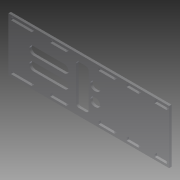
# Autodesk Inventor part: Top_plate2
Saved by Autodesk Inventor 2015 (Build 190159000, 159)
## iProperties
Created: 2015-06-18
Part Number: Top_plate2
Material: Generic
Document SubType Name: Modeling
Designer: Openlab
Density: 1 g/cm^3
Appearance: Polycarbonate - Clear
Author: Openlab
Autodesk Inventor part; units mm, degrees
ref_plane "YZ Plane" through (0, 0, 0) normal (1, 0, 0) x (0, 1, 0)
ref_plane "XZ Plane" through (0, 0, 0) normal (0, 1, 0) x (-1, 0, 0)
ref_plane "XY Plane" through (0, 0, 0) normal (0, 0, 1) x (1, 0, 0)
sketch "Sketch1" plane through (0, 0, 0) normal (0, 1, 0) x (-1, 0, 0)
  line L0 (37.25, -2.25) -> (24.75, -2.25) construction
  line L1 (24.75, -2.25) -> (24.75, -14.75) construction
  line L2 (24.75, -14.75) -> (37.25, -14.75) construction
  line L3 (37.25, -14.75) -> (37.25, -2.25) construction
  line L4 (56.9183, -8.5) -> (8.3915, -8.5) construction
  line L5 (0, -17) -> (105, -17) construction
  line L6 (0, 0) -> (0, -51) construction
  line L7 (0, -34) -> (105, -34) construction
  line L8 (105, -51) -> (105, 0) construction
  line L9 (31, 19) -> (31, -51) construction
  line L10 (56.8064, -25.5) -> (17, -25.5) construction
  line L11 (24.75, -19.25) -> (24.75, -31.75) construction
  line L12 (37.25, -19.25) -> (24.75, -19.25) construction
  line L13 (37.25, -31.75) -> (37.25, -19.25) construction
  line L14 (24.75, -31.75) -> (37.25, -31.75) construction
  line L15 (24.75, -36.25) -> (24.75, -48.75) construction
  line L16 (37.25, -36.25) -> (24.75, -36.25) construction
  line L17 (37.25, -48.75) -> (37.25, -36.25) construction
  line L18 (24.75, -48.75) -> (37.25, -48.75) construction
  line L19 (56.3008, -42.5) -> (16.5498, -42.5) construction
  arc A0 (53.45, -12) -> (53.45, -22) centre (53.45, -17) ccw
  arc A1 (92, -22) -> (92, -12) centre (92, -17) ccw
  arc A2 (53.45, -29) -> (53.45, -39) centre (53.45, -34) ccw
  arc A3 (92, -39) -> (92, -29) centre (92, -34) ccw
  line L20 (53.45, -12) -> (92, -12)
  line L21 (53.45, -22) -> (92, -22)
  line L22 (53.45, -29) -> (92, -29)
  line L23 (53.45, -39) -> (92, -39)
  arc A4 (16.15, -39) -> (16.15, -29) centre (16.15, -34) ccw
  line L24 (103.5, -49.5) -> (103.5, -1.5) construction
  line L25 (1.5, -1.5) -> (1.5, -49.5) construction
  arc A5 (14, -29) -> (14, -39) centre (14, -34) ccw
  arc A6 (14, -12) -> (14, -22) centre (14, -17) ccw
  line L26 (16.15, -39) -> (14, -39)
  line L27 (14, -29) -> (16.15, -29)
  line L28 (14, -22) -> (16.15, -22)
  line L29 (16.15, -12) -> (14, -12)
  arc A7 (16.15, -22) -> (16.15, -12) centre (16.15, -17) ccw
  arc A8 (96.5, -51) -> (93, -47.5) centre (93, -51) ccw construction
  arc A9 (53.45, -47.5) -> (49.95, -51) centre (53.45, -51) ccw construction
  arc A10 (97.7697, -49.5) -> (93, -46) centre (93, -51) ccw construction
  line L30 (93, -46) -> (53.45, -46) construction
  line L31 (96.5, -51) -> (105, -51) construction
  line L32 (93, -47.5) -> (53.45, -47.5) construction
  line L33 (105, -49.5) -> (97.7697, -49.5) construction
  arc A11 (53.45, -46) -> (48.6803, -49.5) centre (53.45, -51) ccw construction
  arc A12 (48.6803, -1.5) -> (53.45, -5) centre (53.45, 0) ccw construction
  arc A13 (49.95, 0) -> (53.45, -3.5) centre (53.45, 0) ccw construction
  line L34 (93, -3.5) -> (53.45, -3.5) construction
  line L35 (93, -5) -> (53.45, -5) construction
  line L36 (97.7697, -1.5) -> (105, -1.5) construction
  line L37 (105, 0) -> (96.5, 0) construction
  arc A14 (93, -3.5) -> (96.5, 0) centre (93, 0) ccw construction
  arc A15 (93, -5) -> (97.7697, -1.5) centre (93, 0) ccw construction
  arc A16 (16.65, -51) -> (13.15, -47.5) centre (13.15, -51) ccw construction
  arc A17 (12, -47.5) -> (8.5, -51) centre (12, -51) ccw construction
  line L38 (13.15, -46) -> (12, -46) construction
  line L39 (13.15, -47.5) -> (12, -47.5) construction
  arc A18 (12, -46) -> (7.2303, -49.5) centre (12, -51) ccw construction
  arc A19 (17.9197, -49.5) -> (13.15, -46) centre (13.15, -51) ccw construction
  line L40 (48.6803, -49.5) -> (17.9197, -49.5) construction
  line L41 (7.2303, -49.5) -> (0, -49.5) construction
  line L42 (0, -51) -> (8.5, -51) construction
  line L43 (16.65, -51) -> (49.95, -51) construction
  line L44 (13.15, -5) -> (12, -5) construction
  line L45 (13.15, -3.5) -> (12, -3.5) construction
  arc A20 (8.5, 0) -> (12, -3.5) centre (12, 0) ccw construction
  arc A21 (13.15, -3.5) -> (16.65, 0) centre (13.15, 0) ccw construction
  arc A22 (7.2303, -1.5) -> (12, -5) centre (12, 0) ccw construction
  arc A23 (13.15, -5) -> (17.9197, -1.5) centre (13.15, 0) ccw construction
  line L46 (49.95, 0) -> (16.65, 0) construction
  line L47 (8.5, 0) -> (0, 0) construction
  line L48 (0, -1.5) -> (7.2303, -1.5) construction
  line L49 (17.9197, -1.5) -> (48.6803, -1.5) construction
  line L50 (-74, 2) -> (-74, -53)
  line L51 (120, -53) -> (120, 2)
  arc A24 (38.75, -4.25) -> (35.25, -0.75) centre (35.25, -4.25) ccw
  arc A25 (26.75, -0.75) -> (23.25, -4.25) centre (26.75, -4.25) ccw
  arc A26 (35.25, -50.25) -> (38.75, -46.75) centre (35.25, -46.75) ccw
  arc A27 (23.25, -46.75) -> (26.75, -50.25) centre (26.75, -46.75) ccw
  line L52 (38.75, -4.25) -> (38.75, -46.75)
  line L53 (35.25, -0.75) -> (26.75, -0.75)
  line L54 (23.25, -4.25) -> (23.25, -46.75)
  line L55 (26.75, -50.25) -> (35.25, -50.25)
  line L56 (120, -53) -> (120, -56)
  line L57 (-74, -56) -> (-74, -53)
  line L58 (120, 2) -> (120, 5)
  line L59 (-74, 5) -> (-74, 2)
  line L60 (51, -56) -> (51, -53)
  line L61 (11, -56) -> (11, -53)
  line L62 (71, -56) -> (71, -53)
  line L63 (94, -53) -> (94, -56)
  line L64 (-9, -53) -> (-9, -56)
  line L65 (-59, -56) -> (-59, -53)
  line L66 (94, 2) -> (94, 5)
  line L67 (71, 2) -> (71, 5)
  line L68 (51, 2) -> (51, 5)
  line L69 (11, 2) -> (11, 5)
  line L70 (-9, 2) -> (-9, 5)
  line L71 (-59, 2) -> (-59, 5)
  line L72 (120, -56) -> (123, -56)
  line L73 (123, -56) -> (123, 5)
  line L74 (123, 5) -> (120, 5)
  line L75 (-74, 5) -> (-77, 5)
  line L76 (-77, 5) -> (-77, -56)
  line L77 (-77, -56) -> (-74, -56)
  line L78 (123, -56) -> (123, -59)
  line L79 (123, -59) -> (-77, -59)
  line L80 (-77, -59) -> (-77, -56)
  line L81 (123, 5) -> (123, 8)
  line L82 (123, 8) -> (-77, 8)
  line L83 (-77, 8) -> (-77, 5)
  line L84 (120, -56) -> (94, -56)
  line L85 (71, -56) -> (51, -56)
  line L86 (11, -56) -> (-9, -56)
  line L87 (-59, -56) -> (-74, -56)
  line L88 (-59, -53) -> (-74, -53)
  line L89 (-9, -53) -> (11, -53)
  line L90 (51, -53) -> (71, -53)
  line L91 (94, -53) -> (120, -53)
  line L92 (120, 5) -> (94, 5)
  line L93 (120, 2) -> (94, 2)
  line L94 (71, 2) -> (51, 2)
  line L95 (71, 5) -> (51, 5)
  line L96 (11, 2) -> (-9, 2)
  line L97 (11, 5) -> (-9, 5)
  line L98 (-59, 2) -> (-74, 2)
  line L99 (-59, 5) -> (-74, 5)
  line L100 (-24, -53) -> (-39, -53)
  line L101 (-39, -53) -> (-39, -56)
  line L102 (-39, -56) -> (-24, -56)
  line L103 (-24, -56) -> (-24, -53)
  line L104 (-24, 5) -> (-39, 5)
  line L105 (-39, 5) -> (-39, 2)
  line L106 (-39, 2) -> (-24, 2)
  line L107 (-24, 2) -> (-24, 5)
  point P0 (31, -8.5)
  point P1 (31, -42.5)
  point P2 (31, -25.5)
  dimension "d0" = 12.5
  dimension "d1" = 12.5
  dimension "d2" = 17
  dimension "d3" = 31
  dimension "d4" = 105
  dimension "d5" = 17
  dimension "d6" = 17
  dimension "d7" = 10
  dimension "d8" = 1.5
  dimension "d9" = 1.5
  dimension "d10" = 5
  dimension "d11" = 1.5
  dimension "d12" = 1.5
  dimension "d13" = 1.5
  dimension "d14" = 17
  dimension "d15" = 17
  dimension "d16" = 12
  dimension "d17" = 13
  dimension "d19" = 11.6
  dimension "d20" = 8.6
  dimension "d21" = 12
  dimension "d24" = 15
  dimension "d28" = 2
  dimension "d29" = 2
  dimension "d30" = 7
  dimension "d31" = 2
  dimension "d32" = 2
  dimension "d38" = 40
  dimension "d39" = 20
  dimension "d40" = 23
  dimension "d42" = 20
  dimension "d44" = 3
  dimension "d46" = 200
  dimension "d48" = 29
  dimension "d50" = 3
  dimension "d51" = 3
  dimension "d53" = 5
  dimension "d55" = 3
  dimension "d56" = 3
  dimension "d57" = 3
  dimension "d60" = 15
  dimension "d61" = 15
  dimension "d62" = 15
  dimension "d63" = 20
  dimension "d64" = 14
  dimension "d65" = 22.45
  dimension "d66" = 10.5
  constraints: 216 end point, 56 point on circle, 42 collinear, 32 point on line, 32 tangent, 28 centre point, 28 parallel, 27 perpendicular, 24 equal radius, 15 horizontal, 11 vertical alignment, 10 coincident, 9 horizontal alignment, 5 vertical, 10 other
  measures "d0" distance of L2.end L1.end
  measures "d1" distance of L0.end L1.end
  measures "d2" distance between parallel lines of L10 L4
  measures "d3" distance between parallel lines of L6 L9
  measures "d4" distance between parallel lines of L6 L8
  measures "d5" distance between parallel lines of L19 L10
  measures "d6" distance between parallel lines of L5 L7
  measures "d7" diameter of A0
  measures "d8" distance between parallel lines of L6 L25
  measures "d9" distance between parallel lines of L8 L24
  measures "d10" radius of A4
  measures "d11" radial gap between concentric circles of A8 A10
  measures "d12" distance between parallel lines of L37 L36
  measures "d13" distance between parallel lines of L41 L42
  measures "d14" distance between parallel lines of L7 L42
  measures "d15" distance between parallel lines of L47 L5
  measures "d16" distance from line of A8.centre L8
  measures "d17" distance from line of L8 A3.centre
  measures "d19" distance from line of A19.centre L15
  measures "d20" distance from line of A4.centre L15
  measures "d21" distance from line of L6 A22.centre
  measures "d24" distance between parallel lines of L8 L51
  measures "d28" distance from line of L1 A25.centre
  measures "d29" distance from line of A25.centre L0
  measures "d30" diameter of A25
  measures "d31" distance from line of L17 A26.centre
  measures "d32" distance from line of L18 A26.centre
  measures "d38" distance between parallel lines of L61 L60
  measures "d39" distance between parallel lines of L62 L60
  measures "d40" distance between parallel lines of L62 L63
  measures "d42" distance between parallel lines of L64 L61
  measures "d44" distance of L56.end L72.end
  measures "d46" distance between parallel lines of L76 L73
  measures "d48" distance between parallel lines of L63 L73
  measures "d50" distance of L72.end L78.end
  measures "d51" distance of L73.end L81.end
  measures "d53" distance between parallel lines of L72 L31
  measures "d55" distance between parallel lines of L90 L85
  measures "d56" distance of L67.start L67.end
  measures "d57" distance between parallel lines of L76 L50
  measures "d60" distance between parallel lines of L57 L65
  measures "d61" distance between parallel lines of L103 L64
  measures "d62" distance of L101.end L102.end
  measures "d63" distance between parallel lines of L65 L101
  measures "d64" distance of L5.start A6.centre
  measures "d65" distance from line of L9 A11.centre
  measures "d66" distance between parallel lines of L89 L19
extrude "Extrusion2" add sketch "Sketch1" along normal blind 3 contours L98 L71 L99 L75 L83 L82 L81 L74 L92 L66 L93 L51 L91 L63 L84 L72 L78 L79 L80 L77 L87 L65 L88 L50 | L50 L57 L77 L76 L75 L59 | L73 L72 L56 L51 L58 L74
body "Solid2"
